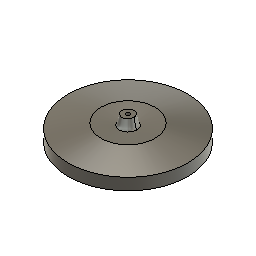
impeller v0 (Autodesk Fusion 360 design; units mm, degrees)
Autodesk Fusion 360 part; units mm, degrees
sketch "Sketch1" plane through (0, 0, 0) normal (0, 0, 1) x (1, 0, 0)
  line L0 (0, 0) -> (34.55, 0)
  line L1 (34.55, 0) -> (34.55, 6.8)
  line L2 (15.6, 0) -> (15.6, 9.67) construction
  line L3 (34.55, 6.8) -> (15.6, 9.67)
  line L4 (5.05, 0) -> (5.05, 8.6) construction
  line L5 (15.6, 9.67) -> (5.05, 8.6)
  line L6 (0, 0) -> (0, 14.12)
  line L7 (0, 14.12) -> (3.475, 14.12)
  spline S0 degree 2 poles (3.475, 14.12) (4.5, 9.5) (5.05, 8.6) knots 0 0 0 0.575587 0.575587 0.575587 weights 1 2.082456 1
  line L8 (3.125, 0) -> (3.125, 5.7)
  line L9 (3.125, 5.7) -> (0, 5.7)
  line L10 (13.66, 0) -> (13.66, 1.45) construction
  spline S1 degree 2 poles (3.125, 5.7) (6, 1.5) (13.66, 1.45) knots 0 0 0 1.170983 1.170983 1.170983
  line L11 (13.66, 1.45) -> (14.4767, 0)
  line L12 (1.16, 0) -> (1.16, 14.12)
  dimension "d1" = 34.55
  dimension "d2" = 6.8
  dimension "d3" = 9.67
  dimension "d4" = 15.6
  dimension "d5" = 8.6
  dimension "d6" = 5.05
  dimension "d7" = 14.12
  dimension "d8" = 3.475
  dimension "d9" = 3.125
  dimension "d10" = 5.7
  dimension "d11" = 1.45
  dimension "d12" = 13.66
  dimension "d13" = 1.16
  constraint coincident L0.start L6.start
  constraint horizontal L0
  constraint perpendicular L0 L1
  constraint coincident L0 L2.start
  constraint perpendicular L0 L2
  constraint coincident L0 L4.start
  constraint perpendicular L0 L4
  constraint perpendicular L0 L6
  constraint perpendicular L6 L7
  constraint coincident L0 L8.start
  constraint perpendicular L0 L8
  constraint coincident L6 L9.end
  constraint perpendicular L6 L9
  constraint coincident L0 L10.start
  constraint perpendicular L0 L10
  constraint coincident L0 L11.end
  constraint coincident L0 L12.start
  constraint perpendicular L0 L12
  constraint coincident L7 L12.end
  measures "d1" distance of L0.start L0.end
  measures "d2" distance of L0.end L1.end
  measures "d3" distance of L2.start L2.end
  measures "d4" distance of L0.start L2
  measures "d5" distance of L4.start L4.end
  measures "d6" distance of L0.start L4
  measures "d7" distance of L0.start L6.end
  measures "d8" distance of L6.end L7.end
  measures "d9" distance of L6 L8
  measures "d10" distance of L8.start L8.end
  measures "d11" distance of L10.start L10.end
  measures "d12" distance of L6 L10
  measures "d13" distance of L6 L12
revolve "Revolve1" add sketch "Sketch1" angle 360 about axis through (0, 0, 0) along (0, 1, 0) contours L0 L8 L9 L12 | L0 L1 L3 L5 L7 S0 L9 S1 L11 L12
sketch "Sketch2" plane through (0, 0, 0) normal (0, -1, 0) x (1, 0, 0)
  circle A0 centre (0, 0) radius 3.125
  circle A1 centre (0, 0) radius 1.16
  line L0 (1, 2.9607) -> (1, 14.4421)
  circle A2 centre (0, 0) radius 34.55
  circle A3 centre (0, 0) radius 14.4767
  line L1 (-1, 14.4421) -> (-1, 2.9607)
  line L2 (0, 3.125) -> (0, 14.4767) construction
  line L3 (0, 0) -> (0, 3.125) construction
  dimension "d15" = 2
  constraint coincident A0 L0.start
  constraint vertical L0
  constraint coincident A3 L1.start
  constraint coincident A0 L1.end
  constraint parallel L0 L1
  constraint coincident A0 L2.start
  constraint coincident A3 L2.end
  constraint parallel L0 L2
  constraint coincident A0.centre A1.centre
  constraint vertical L3
  constraint symmetric L0 L1 L2
  constraint coincident L0.end A3
  measures "d15" distance of L0 L1
extrude "Extrude1" add sketch "Sketch2" against normal blind 7 contours A0 L0 A3 L1 picked at (-0.5123, 10.6778)
pattern_circular "C-Pattern1" count 4 over 360 about axis through (0, 5.7, 0) along (0, -1, 0) of "Extrude1"
equation "d1 = ( 69.1 / 2 ) * 1 mm"
equation "d4 = ( 31.2 / 2 ) * 1 mm"
equation "d6 = ( 10.1 / 2 ) * 1 mm"
equation "d8 = ( 6.95 / 2 ) * 1 mm"
equation "d9 = ( 6.25 / 2 ) * 1 mm"
equation "d12 = ( 27.32 / 2 ) * 1 mm"
equation "d13 = ( 2.32 / 2 ) * 1 mm"
